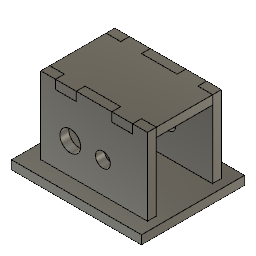
Motor bracket v1 (Autodesk Fusion 360 archive; units mm, degrees)
design "penis"
Autodesk Fusion 360 part; units mm, degrees
sketch "Sketch1" plane through (0, 0, 0) normal (0, 0, 1) x (1, 0, 0)
  line L0 (-34.5, 9.5) -> (34.5, 9.5)
  line L1 (34.5, 9.5) -> (34.5, -9.5)
  line L2 (34.5, -9.5) -> (-34.5, -9.5)
  line L3 (-34.5, -9.5) -> (-34.5, 9.5)
  line L4 (-34.5, 9.5) -> (34.5, -9.5) construction
  line L5 (34.5, 9.5) -> (-34.5, -9.5) construction
  line L6 (-34.5, -9.5) -> (34.5, -9.5)
  line L7 (34.5, -9.5) -> (34.5, -12.4)
  line L8 (34.5, -12.4) -> (-34.5, -12.4)
  line L9 (-34.5, -12.4) -> (-34.5, -9.5)
  line L10 (-34.5, 9.5) -> (34.5, 9.5)
  line L11 (34.5, 9.5) -> (34.5, 12.4)
  line L12 (34.5, 12.4) -> (-34.5, 12.4)
  line L13 (-34.5, 12.4) -> (-34.5, 9.5)
  line L14 (-34.5, -12.4) -> (34.5, -12.4)
  line L15 (34.5, -12.4) -> (34.5, -17.4)
  line L16 (34.5, -17.4) -> (-34.5, -17.4)
  line L17 (-34.5, -17.4) -> (-34.5, -12.4)
  line L18 (-34.5, 12.4) -> (34.5, 12.4)
  line L19 (34.5, 12.4) -> (34.5, 17.4)
  line L20 (34.5, 17.4) -> (-34.5, 17.4)
  line L21 (-34.5, 17.4) -> (-34.5, 12.4)
  line L22 (-34.5, 17.4) -> (-34.5, -17.4)
  line L23 (-34.5, -17.4) -> (-39.5, -17.4)
  line L24 (-39.5, -17.4) -> (-39.5, 17.4)
  line L25 (-39.5, 17.4) -> (-34.5, 17.4)
  line L26 (34.5, 17.4) -> (34.5, -17.4)
  line L27 (34.5, -17.4) -> (39.5, -17.4)
  line L28 (39.5, -17.4) -> (39.5, 17.4)
  line L29 (39.5, 17.4) -> (34.5, 17.4)
  dimension "d1" = 69
  dimension "d2" = 19
  dimension "d3" = 2.9
  dimension "d4" = 2.9
  dimension "d5" = 5
  dimension "d6" = 5
  dimension "d7" = 5
  dimension "d8" = 5
  constraint horizontal L0
  constraint perpendicular L0 L1
  constraint parallel L0 L2
  constraint parallel L1 L3
  constraint coincident L4 origin
  constraint coincident L5 origin
  constraint perpendicular L6 L7
  constraint parallel L6 L8
  constraint parallel L7 L9
  constraint perpendicular L10 L11
  constraint parallel L10 L12
  constraint parallel L11 L13
  constraint perpendicular L14 L15
  constraint parallel L14 L16
  constraint parallel L15 L17
  constraint perpendicular L18 L19
  constraint parallel L18 L20
  constraint parallel L19 L21
  constraint perpendicular L22 L23
  constraint parallel L22 L24
  constraint parallel L23 L25
  constraint perpendicular L26 L27
  constraint parallel L26 L28
  constraint parallel L27 L29
  measures "d1" distance of L1.end L2.end
  measures "d2" distance of L0.end L1.end
  measures "d3" distance of L2.end L8.end
  measures "d4" distance of L0.start L12.end
  measures "d5" distance of L8.end L16.end
  measures "d6" distance of L12.end L20.end
  measures "d7" distance of L20.end L24.end
  measures "d8" distance of L19.end L28.end
extrude "Extrude1" add sketch "Sketch1" along normal blind 3 contours L0 L1 L2 L3 L6 L10 L22 L26 | L3 L9 L13 L17 L21 L22 L23 L24 L25 | L1 L7 L11 L15 L19 L26 L27 L28 L29 | L12 L18 L19 L20 L21 L22 L26 | L8 L14 L15 L16 L17 L22 L26 makes body 1
sketch "Sketch2" plane through (0, -9.5, 0) normal (0, -1, 0) x (1, 0, 0)
  line L0 (-34.5, 0) -> (34.5, 0)
  line L1 (34.5, 0) -> (34.5, 3)
  line L2 (34.5, 3) -> (-34.5, 3)
  line L3 (-34.5, 3) -> (-34.5, 0)
  line L4 (-34.5, 3) -> (34.5, 3)
  line L5 (34.5, 3) -> (34.5, 26)
  line L6 (34.5, 26) -> (-34.5, 26)
  line L7 (-34.5, 26) -> (-34.5, 3)
  line L8 (-34.5, 26) -> (-34.5, 3)
  line L9 (-34.5, 3) -> (-24.5, 3)
  line L10 (-24.5, 3) -> (-24.5, 26) construction
  line L11 (-24.5, 26) -> (-34.5, 26)
  line L12 (34.5, 3) -> (-34.5, 3) construction
  line L13 (-34.5, 3) -> (-34.5, 13.5) construction
  line L14 (-34.5, 13.5) -> (34.5, 13.5) construction
  line L15 (34.5, 13.5) -> (34.5, 3) construction
  line L16 (-24.5, 13.5) -> (-13.5, 13.5) construction
  circle A0 centre (-13.5, 13.5) radius 2.5
  circle A1 centre (-24.5, 13.5) radius 3.5
  line L17 (-13.5, 13.5) -> (1.5, 13.5) construction
  line L18 (1.5, 13.5) -> (1.5, 3)
  line L19 (1.5, 13.5) -> (1.5, 26)
  line L20 (1.5, 3) -> (1.5, 0)
  dimension "d11" = 23
  dimension "d12" = 10
  dimension "d13" = 10.5
  dimension "d14" = 11
  dimension "d15" = 5
  dimension "d16" = 7
  dimension "d17" = 15
  constraint perpendicular L4 L5
  constraint parallel L4 L6
  constraint parallel L5 L7
  constraint coincident L1.end L2.start
  constraint perpendicular L1 L4
  constraint coincident L2.end L3.start
  constraint perpendicular L8 L9
  constraint parallel L8 L10
  constraint parallel L9 L11
  constraint perpendicular L12 L13
  constraint parallel L12 L14
  constraint parallel L13 L15
  constraint coincident L10 L16.start
  constraint coincident L14 L16.start
  constraint perpendicular L10 L16
  constraint coincident L16.end A0.centre
  constraint coincident L16.start A1.centre
  constraint parallel L14 L17
  constraint coincident L4 L18.end
  constraint perpendicular L4 L18
  constraint coincident L6 L19.end
  constraint perpendicular L6 L19
  constraint coincident L0 L20.end
  constraint perpendicular L0 L20
  measures "d11" distance of L2.end L6.end
  measures "d12" distance of L6.end L10.end
  measures "d13" distance of L1.end L14.end
  measures "d14" distance of L16.start L16.end
  measures "d15" diameter of A0
  measures "d16" diameter of A1
  measures "d17" distance of L16.end L17.end
extrude "Extrude2" add sketch "Sketch2" along normal blind 3 separate body contours L0 L2 L3 L4 L9 L20 | L2 L4 L6 L7 L8 L9 L11 L18 L19 makes body 2
sketch "Sketch3" plane through (0, 0, 26) normal (0, 0, 1) x (-1, 0, 0)
  line L0 (-1.5, 9.5) -> (34.5, 9.5)
  line L1 (34.5, 9.5) -> (34.5, 12.5)
  line L2 (34.5, 12.5) -> (-1.5, 12.5)
  line L3 (-1.5, 12.5) -> (-1.5, 9.5)
  line L4 (-1.5, 12.5) -> (3.5, 12.5)
  line L5 (3.5, 12.5) -> (3.5, 9.5)
  line L6 (3.5, 9.5) -> (-1.5, 9.5)
  line L7 (-1.5, 9.5) -> (-1.5, 12.5)
  line L8 (34.5, 12.5) -> (29.5, 12.5)
  line L9 (29.5, 12.5) -> (29.5, 9.5)
  line L10 (29.5, 9.5) -> (34.5, 9.5)
  line L11 (34.5, 9.5) -> (34.5, 12.5)
  line L12 (3.5, 9.5) -> (3.5, 12.5)
  line L13 (3.5, 12.5) -> (10.5, 12.5)
  line L14 (10.5, 12.5) -> (10.5, 9.5)
  line L15 (10.5, 9.5) -> (3.5, 9.5)
  line L16 (29.5, 12.5) -> (29.5, 9.5)
  line L17 (29.5, 9.5) -> (22.5, 9.5)
  line L18 (22.5, 9.5) -> (22.5, 12.5)
  line L19 (22.5, 12.5) -> (29.5, 12.5)
  dimension "d20" = 5
  dimension "d21" = 5
  dimension "d22" = 7
  dimension "d23" = 7
  constraint horizontal L4
  constraint vertical L5
  constraint horizontal L6
  constraint vertical L7
  constraint coincident L2.end L3.start
  constraint horizontal L8
  constraint vertical L9
  constraint horizontal L10
  constraint vertical L11
  constraint coincident L1.end L2.start
  constraint perpendicular L12 L13
  constraint parallel L12 L14
  constraint parallel L13 L15
  constraint perpendicular L16 L17
  constraint parallel L16 L18
  constraint parallel L17 L19
  measures "d20" distance of L2.end L4.end
  measures "d21" distance of L1.end L8.end
  measures "d22" distance of L5.end L14.end
  measures "d23" distance of L8.end L18.end
extrude "Extrude3" add sketch "Sketch3" along normal blind 3 contours L0 L2 L3 L4 L5 L6 L7 L12 | L0 L2 L14 L18 | L0 L1 L2 L8 L9 L10 L11 L16 bodies 2
copy_body "CopyPasteBodies1" bodies 2 makes body 3
move_body "Move1" bodies 3 to x (1, 0, 0) y (0, 1, 0) z (0, 0, 1) at (0, 22, 0)
sketch "Sketch4" plane through (0, 0, 26) normal (0, 0, 1) x (-1, 0, 0)
  line L0 (10.5, 9.5) -> (10.5, 12.5)
  line L1 (10.5, 12.5) -> (3.5, 12.5)
  line L2 (3.5, 12.5) -> (3.5, 9.5)
  line L3 (3.5, 9.5) -> (10.5, 9.5)
  line L4 (29.5, 9.5) -> (29.5, 12.5)
  line L5 (29.5, 12.5) -> (22.5, 12.5)
  line L6 (22.5, 12.5) -> (22.5, 9.5)
  line L7 (22.5, 9.5) -> (29.5, 9.5)
  line L8 (29.5, -12.5) -> (29.5, -9.5)
  line L9 (29.5, -9.5) -> (22.5, -9.5)
  line L10 (22.5, -9.5) -> (22.5, -12.5)
  line L11 (22.5, -12.5) -> (29.5, -12.5)
  line L12 (10.5, -12.5) -> (10.5, -9.5)
  line L13 (10.5, -9.5) -> (3.5, -9.5)
  line L14 (3.5, -9.5) -> (3.5, -12.5)
  line L15 (3.5, -12.5) -> (10.5, -12.5)
  line L16 (-1.5, 9.5) -> (3.5, 9.5)
  line L17 (3.5, 9.5) -> (3.5, 12.5)
  line L18 (3.5, 12.5) -> (-1.5, 12.5)
  line L19 (-1.5, 12.5) -> (-1.5, 9.5)
  line L20 (-1.5, -12.5) -> (3.5, -12.5)
  line L21 (3.5, -12.5) -> (3.5, -9.5)
  line L22 (3.5, -9.5) -> (-1.5, -9.5)
  line L23 (-1.5, -9.5) -> (-1.5, -12.5)
  line L24 (29.5, -9.5) -> (29.5, -12.5)
  line L25 (29.5, -12.5) -> (34.5, -12.5)
  line L26 (34.5, -12.5) -> (34.5, -9.5)
  line L27 (34.5, -9.5) -> (29.5, -9.5)
  line L28 (29.5, 12.5) -> (29.5, 9.5)
  line L29 (29.5, 9.5) -> (34.5, 9.5)
  line L30 (34.5, 9.5) -> (34.5, 12.5)
  line L31 (34.5, 12.5) -> (29.5, 12.5)
  line L32 (-1.5, 9.5) -> (34.5, 9.5)
  line L33 (34.5, 9.5) -> (34.5, -9.5)
  line L34 (34.5, -9.5) -> (-1.5, -9.5)
  line L35 (-1.5, -9.5) -> (-1.5, 9.5)
  constraint horizontal L32
  constraint vertical L33
  constraint horizontal L34
  constraint vertical L35
  constraint coincident L26.end L27.start
  constraint coincident L16.start L19.end
extrude "Extrude4" add sketch "Sketch4" along normal blind 3 separate body contours L0 L1 L2 L3 L17 L32 | L3 L7 L9 L13 L16 L22 L27 L29 L32 L33 L34 L35 | L4 L5 L6 L7 L28 L32 | L12 L13 L14 L15 L21 L34 | L8 L9 L10 L11 L24 L34 makes body 4
sketch "Sketch5" plane through (0, -12.4, 0) normal (0, 1, 0) x (-1, 0, 0)
  line L0 (-34.5, 0) -> (34.5, 0)
  line L1 (34.5, 0) -> (34.5, 3)
  line L2 (34.5, 3) -> (-34.5, 3)
  line L3 (-34.5, 3) -> (-34.5, 0)
  line L4 (-1.5, 0) -> (-1.5, 29)
  line L5 (-1.5, 29) -> (-1.5, 0)
  line L6 (-1.5, 0) -> (-1.5, 3)
  line L7 (-1.5, 3) -> (-1.4, 3)
  line L8 (-1.4, 3) -> (-1.4, 0)
  line L9 (-1.4, 0) -> (-1.5, 0)
  dimension "d28" = 0.1
  constraint perpendicular L6 L7
  constraint parallel L6 L8
  constraint parallel L7 L9
  constraint coincident L2 L6.end
  constraint coincident L4 L6.end
  constraint perpendicular L2 L6
  constraint coincident L4.start L5.end
  measures "d28" distance of L4.start L8.end
extrude "Extrude5" add sketch "Sketch5" along normal blind 29.8 contours L0 L2 L3 L4 L5 L6 | L0 L2 L4 L5 L6 L7 L8 L9 bodies 1
extrude "Extrude6" cut 1 faces at (39.5, -5.8, 2) along direction (-1, 0, 0) blind 35.1 on bodies 1 bodies 1
equation "d14 = 3.5 mm + 2.5 mm + 5 mm"
equation "d31 = -38.10 mm + 3 mm"
